Autodesk Inventor part; units mm, degrees
(part 4 of 4)
sketch "Эскиз15" plane through (0, 0, 5) normal (0, 0, 1) x (1, 0, 0)
  circle A0 centre (-47.4326, -62.0164) radius 1.6 projected
  circle A1 centre (-37.1084, -66.6437) radius 1.6 projected
  circle A2 centre (-32.4811, -56.3196) radius 1.6 projected
  circle A3 centre (-39.9568, -59.168) radius 2.5 projected
  circle A4 centre (-42.8052, -51.6922) radius 1.6 projected
  arc A5 (-41.4259, -46.9885) -> (-28.2942, -62.9735) centre (-39.9568, -59.168) ccw projected
  line L0 (-28.085, -62.2597) -> (-28.2942, -62.9735) projected
  line L1 (-27.9195, -61.5344) -> (-28.085, -62.2597) projected
  line L2 (-27.7675, -61.2078) -> (-27.9195, -61.5344) projected
  line L3 (-27.6559, -61.0885) -> (-27.7675, -61.2078) projected
  line L4 (-27.5511, -61.0052) -> (-27.6559, -61.0885) projected
  line L5 (-27.4498, -60.9413) -> (-27.5511, -61.0052) projected
  line L6 (-27.3508, -60.8903) -> (-27.4498, -60.9413) projected
  line L7 (-27.1571, -60.815) -> (-27.3508, -60.8903) projected
  line L8 (-26.9672, -60.7651) -> (-27.1571, -60.815) projected
  line L9 (-26.78, -60.734) -> (-26.9672, -60.7651) projected
  line L10 (-26.5947, -60.7178) -> (-26.78, -60.734) projected
  line L11 (-26.2284, -60.7215) -> (-26.5947, -60.7178) projected
  line L12 (-25.8656, -60.755) -> (-26.2284, -60.7215) projected
  line L13 (-25.4958, -60.7256) -> (-25.8656, -60.755) projected
  line L14 (-25.1221, -60.6541) -> (-25.4958, -60.7256) projected
  line L15 (-24.7463, -60.5502) -> (-25.1221, -60.6541) projected
  line L16 (-24.3693, -60.4182) -> (-24.7463, -60.5502) projected
  line L17 (-23.9923, -60.2602) -> (-24.3693, -60.4182) projected
  line L18 (-23.616, -60.0777) -> (-23.9923, -60.2602) projected
  line L19 (-23.2412, -59.8717) -> (-23.616, -60.0777) projected
  line L20 (-22.8687, -59.6431) -> (-23.2412, -59.8717) projected
  line L21 (-22.4992, -59.3924) -> (-22.8687, -59.6431) projected
  line L22 (-22.2246, -59.1902) -> (-22.4992, -59.3924) projected
  line L23 (-22.3522, -57.0445) -> (-22.2246, -59.1902) projected
  line L24 (-22.6489, -56.8763) -> (-22.3522, -57.0445) projected
  line L25 (-23.0454, -56.6711) -> (-22.6489, -56.8763) projected
  line L26 (-23.4424, -56.4882) -> (-23.0454, -56.6711) projected
  line L27 (-23.839, -56.3281) -> (-23.4424, -56.4882) projected
  line L28 (-24.2343, -56.1915) -> (-23.839, -56.3281) projected
  line L29 (-24.6274, -56.0793) -> (-24.2343, -56.1915) projected
  line L30 (-25.0173, -55.9929) -> (-24.6274, -56.0793) projected
  line L31 (-25.4028, -55.9343) -> (-25.0173, -55.9929) projected
  line L32 (-25.7823, -55.9075) -> (-25.4028, -55.9343) projected
  line L33 (-26.153, -55.9222) -> (-25.7823, -55.9075) projected
  line L34 (-26.5093, -55.9985) -> (-26.153, -55.9222) projected
  line L35 (-26.8725, -56.0456) -> (-26.5093, -55.9985) projected
  line L36 (-27.0584, -56.0515) -> (-26.8725, -56.0456) projected
  line L37 (-27.248, -56.0427) -> (-27.0584, -56.0515) projected
  line L38 (-27.4425, -56.0157) -> (-27.248, -56.0427) projected
  line L39 (-27.6437, -55.9639) -> (-27.4425, -56.0157) projected
  line L40 (-27.7481, -55.925) -> (-27.6437, -55.9639) projected
  line L41 (-27.8563, -55.8736) -> (-27.7481, -55.925) projected
  line L42 (-27.9702, -55.8032) -> (-27.8563, -55.8736) projected
  line L43 (-28.0951, -55.698) -> (-27.9702, -55.8032) projected
  line L44 (-28.2847, -55.3917) -> (-28.0951, -55.698) projected
  line L45 (-28.5351, -54.6912) -> (-28.2847, -55.3917) projected
  line L46 (-28.8274, -54.0071) -> (-28.5351, -54.6912) projected
  line L47 (-28.8965, -53.6536) -> (-28.8274, -54.0071) projected
  line L48 (-28.8763, -53.4914) -> (-28.8965, -53.6536) projected
  line L49 (-28.8405, -53.3624) -> (-28.8763, -53.4914) projected
  line L50 (-28.7962, -53.2512) -> (-28.8405, -53.3624) projected
  line L51 (-28.746, -53.1517) -> (-28.7962, -53.2512) projected
  line L52 (-28.6335, -52.977) -> (-28.746, -53.1517) projected
  line L53 (-28.5092, -52.825) -> (-28.6335, -52.977) projected
  line L54 (-28.3761, -52.6897) -> (-28.5092, -52.825) projected
  line L55 (-28.2357, -52.5677) -> (-28.3761, -52.6897) projected
  line L56 (-27.9372, -52.3554) -> (-28.2357, -52.5677) projected
  line L57 (-27.624, -52.1693) -> (-27.9372, -52.3554) projected
  line L58 (-27.3421, -51.9282) -> (-27.624, -52.1693) projected
  line L59 (-27.0818, -51.6507) -> (-27.3421, -51.9282) projected
  line L60 (-26.8388, -51.3457) -> (-27.0818, -51.6507) projected
  line L61 (-26.6114, -51.0173) -> (-26.8388, -51.3457) projected
  line L62 (-26.3993, -50.6679) -> (-26.6114, -51.0173) projected
  line L63 (-26.2021, -50.2991) -> (-26.3993, -50.6679) projected
  line L64 (-26.02, -49.9121) -> (-26.2021, -50.2991) projected
  line L65 (-25.853, -49.5082) -> (-26.02, -49.9121) projected
  line L66 (-25.7014, -49.0882) -> (-25.853, -49.5082) projected
  line L67 (-25.5981, -48.7632) -> (-25.7014, -49.0882) projected
  line L68 (-25.5981, -48.7632) -> (-26.9625, -47.1023) projected
  line L69 (-27.3014, -47.1406) -> (-26.9625, -47.1023) projected
  line L70 (-27.7429, -47.2077) -> (-27.3014, -47.1406) projected
  line L71 (-28.1715, -47.2931) -> (-27.7429, -47.2077) projected
  line L72 (-28.5864, -47.3967) -> (-28.1715, -47.2931) projected
  line L73 (-28.9865, -47.5185) -> (-28.5864, -47.3967) projected
  line L74 (-29.3705, -47.6588) -> (-28.9865, -47.5185) projected
  line L75 (-29.7368, -47.818) -> (-29.3705, -47.6588) projected
  line L76 (-30.0831, -47.9973) -> (-29.7368, -47.818) projected
  line L77 (-30.4059, -48.1987) -> (-30.0831, -47.9973) projected
  line L78 (-30.6971, -48.4284) -> (-30.4059, -48.1987) projected
  line L79 (-30.9405, -48.6995) -> (-30.6971, -48.4284) projected
  line L80 (-31.2067, -48.9511) -> (-30.9405, -48.6995) projected
  line L81 (-31.3536, -49.0652) -> (-31.2067, -48.9511) projected
  line L82 (-31.5122, -49.1695) -> (-31.3536, -49.0652) projected
  line L83 (-31.6854, -49.262) -> (-31.5122, -49.1695) projected
  line L84 (-31.8786, -49.3384) -> (-31.6854, -49.262) projected
  line L85 (-31.986, -49.3683) -> (-31.8786, -49.3384) projected
  line L86 (-32.1037, -49.3902) -> (-31.986, -49.3683) projected
  line L87 (-32.2372, -49.4003) -> (-32.1037, -49.3902) projected
  line L88 (-32.4002, -49.3886) -> (-32.2372, -49.4003) projected
  line L89 (-32.7336, -49.2522) -> (-32.4002, -49.3886) projected
  line L90 (-33.3479, -48.8326) -> (-32.7336, -49.2522) projected
  line L91 (-33.9864, -48.4511) -> (-33.3479, -48.8326) projected
  line L92 (-34.2501, -48.2056) -> (-33.9864, -48.4511) projected
  line L93 (-34.3291, -48.0626) -> (-34.2501, -48.2056) projected
  line L94 (-34.376, -47.9372) -> (-34.3291, -48.0626) projected
  line L95 (-34.4055, -47.8211) -> (-34.376, -47.9372) projected
  line L96 (-34.4234, -47.7112) -> (-34.4055, -47.8211) projected
  line L97 (-34.4351, -47.5037) -> (-34.4234, -47.7112) projected
  line L98 (-34.4238, -47.3077) -> (-34.4351, -47.5037) projected
  line L99 (-34.3956, -47.12) -> (-34.4238, -47.3077) projected
  line L100 (-34.3538, -46.9387) -> (-34.3956, -47.12) projected
  line L101 (-34.237, -46.5916) -> (-34.3538, -46.9387) projected
  line L102 (-34.0931, -46.2568) -> (-34.237, -46.5916) projected
  line L103 (-34.0067, -45.8961) -> (-34.0931, -46.2568) projected
  line L104 (-33.9593, -45.5186) -> (-34.0067, -45.8961) projected
  line L105 (-33.9419, -45.129) -> (-33.9593, -45.5186) projected
  line L106 (-33.951, -44.7298) -> (-33.9419, -45.129) projected
  line L107 (-33.9848, -44.3224) -> (-33.951, -44.7298) projected
  line L108 (-34.0421, -43.9081) -> (-33.9848, -44.3224) projected
  line L109 (-34.1221, -43.488) -> (-34.0421, -43.9081) projected
  line L110 (-34.2244, -43.063) -> (-34.1221, -43.488) projected
  line L111 (-34.3487, -42.6342) -> (-34.2244, -43.063) projected
  line L112 (-34.4561, -42.3105) -> (-34.3487, -42.6342) projected
  line L113 (-36.5363, -41.7688) -> (-34.4561, -42.3105) projected
  line L114 (-36.7879, -41.999) -> (-36.5363, -41.7688) projected
  line L115 (-37.1056, -42.3127) -> (-36.7879, -41.999) projected
  line L116 (-37.4022, -42.6338) -> (-37.1056, -42.3127) projected
  line L117 (-37.677, -42.9614) -> (-37.4022, -42.6338) projected
  line L118 (-37.9291, -43.2952) -> (-37.677, -42.9614) projected
  line L119 (-38.1573, -43.6344) -> (-37.9291, -43.2952) projected
  line L120 (-38.36, -43.9785) -> (-38.1573, -43.6344) projected
  line L121 (-38.5348, -44.327) -> (-38.36, -43.9785) projected
  line L122 (-38.6775, -44.6797) -> (-38.5348, -44.327) projected
  line L123 (-38.7781, -45.0367) -> (-38.6775, -44.6797) projected
  line L124 (-38.8157, -45.3992) -> (-38.7781, -45.0367) projected
  line L125 (-38.8831, -45.7592) -> (-38.8157, -45.3992) projected
  line L126 (-38.935, -45.9378) -> (-38.8831, -45.7592) projected
  line L127 (-39.0019, -46.1155) -> (-38.935, -45.9378) projected
  line L128 (-39.0877, -46.292) -> (-39.0019, -46.1155) projected
  line L129 (-39.1991, -46.4674) -> (-39.0877, -46.292) projected
  line L130 (-39.2684, -46.5547) -> (-39.1991, -46.4674) projected
  line L131 (-39.3507, -46.6417) -> (-39.2684, -46.5547) projected
  line L132 (-39.4528, -46.7283) -> (-39.3507, -46.6417) projected
  line L133 (-39.5916, -46.8146) -> (-39.4528, -46.7283) projected
  line L134 (-39.9414, -46.9002) -> (-39.5916, -46.8146) projected
  line L135 (-40.685, -46.9219) -> (-39.9414, -46.9002) projected
  line L136 (-41.4259, -46.9885) -> (-40.685, -46.9219) projected
  circle A6 centre (-39.9568, -59.168) radius 12.2678
  point P0 (0, 0)
  point P1 (-32.7336, -49.2522)
  point P2 (-28.8274, -54.0071)
  point P3 (-33.9864, -48.4511)
  constraints: 1 centre point, 1 concentric
extrude "Выдавливание14" cut sketch "Эскиз15" against normal blind 10 contours L134 L133 L132 L131 L130 L129 L128 L127 L126 L125 L124 L123 L122 L121 L120 L119 L118 L117 L116 L115 L114 L113 L112 L111 L110 L109 L108 L107 L106 L105 L104 L103 L102 L101 L100 L99 L98 L97 L96 L95 L94 L93 L92 A6 | A6 L44 L43 L42 L41 L40 L39 L38 L37 L36 L35 L34 L33 L32 L31 L30 L29 L28 L27 L26 L25 L24 L23 L22 L21 L20 L19 L18 L17 L16 L15 L14 L13 L12 L11 L10 L9 L8 L7 L6 L5 L4 L3 L2 | L89 L88 L87 L86 L85 L84 L83 L82 L81 L80 L79 L78 L77 L76 L75 L74 L73 L72 L71 L70 L69 L68 L67 L66 L65 L64 L63 L62 L61 L60 L59 L58 L57 L56 L55 L54 L53 L52 L51 L50 L49 L48 L47 A6
sketch "Эскиз16" plane through (0, 0, 5) normal (0, 0, 1) x (1, 0, 0)
  arc A0 (-16.2314, -59.2639) -> (-22.5655, -38.0436) centre (-14.0874, -47.0684) ccw projected
  arc A1 (-22.5655, -38.0436) -> (-25.2878, -36.7337) centre (-28.6703, -47.2467) ccw projected
  arc A2 (-25.2878, -36.7337) -> (-25.9966, -37.559) centre (-14.0874, -47.0684) ccw projected
  arc A3 (-25.9966, -37.559) -> (-24.2901, -40.052) centre (-16.1157, -32.6262) ccw projected
  arc A4 (-24.2901, -40.052) -> (-24.7647, -40.7978) centre (-14.0874, -47.0684) ccw projected
  arc A5 (-24.7647, -40.7978) -> (-27.7458, -40.3078) centre (-28.0294, -51.3479) ccw projected
  arc A6 (-27.7458, -40.3078) -> (-28.1933, -41.2994) centre (-14.0874, -47.0684) ccw projected
  arc A7 (-28.1933, -41.2994) -> (-25.8536, -43.2107) centre (-20.1024, -33.7826) ccw projected
  arc A8 (-25.8536, -43.2107) -> (-26.0988, -44.0599) centre (-14.0874, -47.0684) ccw projected
  arc A9 (-26.0988, -44.0599) -> (-29.0972, -44.4297) centre (-26.2589, -55.1025) ccw projected
  arc A10 (-29.0972, -44.4297) -> (-29.2472, -45.5072) centre (-14.0874, -47.0684) ccw projected
  arc A11 (-29.2472, -45.5072) -> (-26.4639, -46.6819) centre (-23.6018, -36.0154) ccw projected
  arc A12 (-26.4639, -46.6819) -> (-26.4599, -47.5658) centre (-14.0874, -47.0684) ccw projected
  arc A13 (-26.4599, -47.5658) -> (-29.2326, -48.7653) centre (-23.5025, -58.2062) ccw projected
  arc A14 (-29.2326, -48.7653) -> (-29.073, -49.8415) centre (-14.0874, -47.0684) ccw projected
  arc A15 (-29.073, -49.8415) -> (-26.0714, -50.1844) centre (-26.3304, -39.1437) ccw projected
  arc A16 (-26.0714, -50.1844) -> (-25.8186, -51.0314) centre (-14.0874, -47.0684) ccw projected
  arc A17 (-25.8186, -51.0314) -> (-28.1411, -52.9635) centre (-19.9832, -60.4075) ccw projected
  arc A18 (-28.1411, -52.9635) -> (-27.6847, -53.9511) centre (-14.0874, -47.0684) ccw projected
  arc A19 (-27.6847, -53.9511) -> (-24.7081, -53.4345) centre (-28.0671, -42.9139) ccw projected
  arc A20 (-24.7081, -53.4345) -> (-24.2269, -54.1759) centre (-14.0874, -47.0684) ccw projected
  arc A21 (-24.2269, -54.1759) -> (-25.911, -56.6841) centre (-15.9863, -61.5283) ccw projected
  arc A22 (-25.911, -56.6841) -> (-25.1949, -57.5031) centre (-14.0874, -47.0684) ccw projected
  arc A23 (-25.1949, -57.5031) -> (-22.4844, -56.1688) centre (-28.6713, -47.0208) ccw projected
  arc A24 (-22.4844, -56.1688) -> (-21.8138, -56.7447) centre (-14.0874, -47.0684) ccw projected
  arc A25 (-21.8138, -56.7447) -> (-22.723, -59.6257) centre (-11.8356, -61.4775) ccw projected
  arc A26 (-22.723, -59.6257) -> (-21.8052, -60.2097) centre (-14.0874, -47.0684) ccw projected
  arc A27 (-21.8052, -60.2097) -> (-19.5804, -58.1659) centre (-28.094, -51.1315) ccw projected
  arc A28 (-19.5804, -58.1659) -> (-18.7747, -58.5295) centre (-14.0874, -47.0684) ccw projected
  arc A29 (-18.7747, -58.5295) -> (-18.8354, -61.5499) centre (-7.8673, -60.2595) ccw projected
  arc A30 (-18.8354, -61.5499) -> (-17.7902, -61.8518) centre (-14.0874, -47.0684) ccw projected
  arc A31 (-17.7902, -61.8518) -> (-16.2314, -59.2639) centre (-26.3819, -54.913) ccw projected
  circle A32 centre (-9.9505, -53.9158) radius 1.6 projected
  circle A33 centre (-20.9347, -51.2053) radius 1.6 projected
  circle A34 centre (-18.2243, -40.2211) radius 1.6 projected
  circle A35 centre (-7.2401, -42.9315) radius 1.6 projected
  circle A36 centre (-14.0874, -47.0684) radius 2.5 projected
  arc A37 (-27.9195, -61.5344) -> (-28.2847, -55.3917) centre (-39.9568, -59.168) ccw projected
  line L0 (-28.5351, -54.6912) -> (-28.2847, -55.3917) projected
  line L1 (-28.8274, -54.0071) -> (-28.5351, -54.6912) projected
  arc A38 (-28.8274, -54.0071) -> (-32.7336, -49.2522) centre (-39.9568, -59.168) ccw projected
  line L2 (-33.3479, -48.8326) -> (-32.7336, -49.2522) projected
  line L3 (-33.9864, -48.4511) -> (-33.3479, -48.8326) projected
  arc A39 (-33.9864, -48.4511) -> (-39.9414, -46.9002) centre (-39.9568, -59.168) ccw projected
  line L4 (-40.685, -46.9219) -> (-39.9414, -46.9002) projected
  line L5 (-41.4259, -46.9885) -> (-40.685, -46.9219) projected
  arc A40 (-41.4259, -46.9885) -> (-28.2942, -62.9735) centre (-39.9568, -59.168) ccw projected
  line L6 (-28.085, -62.2597) -> (-28.2942, -62.9735) projected
  line L7 (-27.9195, -61.5344) -> (-28.085, -62.2597) projected
  circle A41 centre (-47.4326, -62.0164) radius 1.6 projected
  circle A42 centre (-37.1084, -66.6437) radius 1.6 projected
  circle A43 centre (-32.4811, -56.3196) radius 1.6 projected
  circle A44 centre (-39.9568, -59.168) radius 2.5 projected
  circle A45 centre (-42.8052, -51.6922) radius 1.6 projected
  arc A46 (-28.8099, -64.5599) -> (-28.4537, -63.7509) centre (-39.9568, -59.168) ccw
  arc A47 (-28.4537, -63.7509) -> (-25.4328, -63.7842) centre (-26.8229, -52.8283) ccw
  arc A48 (-25.4328, -63.7842) -> (-25.1404, -62.7363) centre (-39.9568, -59.168) ccw
  arc A49 (-25.1404, -62.7363) -> (-27.7424, -61.201) centre (-32.0008, -71.3907) ccw
  arc A50 (-27.7424, -61.201) -> (-27.6284, -60.3245) centre (-39.9568, -59.168) ccw
  arc A51 (-27.6284, -60.3245) -> (-24.7206, -59.5053) centre (-29.141, -49.3848) ccw
  arc A52 (-24.7206, -59.5053) -> (-24.7353, -58.4175) centre (-39.9568, -59.168) ccw
  arc A53 (-24.7353, -58.4175) -> (-27.6644, -57.6775) centre (-28.8796, -68.6541) ccw
  arc A54 (-27.6644, -57.6775) -> (-27.802, -56.8043) centre (-39.9568, -59.168) ccw
  arc A55 (-27.802, -56.8043) -> (-25.2427, -55.1991) centre (-32.3353, -46.7339) ccw
  arc A56 (-25.2427, -55.1991) -> (-25.5633, -54.1595) centre (-39.9568, -59.168) ccw
  arc A57 (-25.5633, -54.1595) -> (-28.5822, -54.2747) centre (-26.6557, -65.1491) ccw
  arc A58 (-28.5822, -54.2747) -> (-28.9603, -53.4757) centre (-39.9568, -59.168) ccw
  arc A59 (-28.9603, -53.4757) -> (-26.9569, -51.2144) centre (-36.1472, -45.0904) ccw
  arc A60 (-26.9569, -51.2144) -> (-27.5574, -50.3073) centre (-39.9568, -59.168) ccw
  arc A61 (-27.5574, -50.3073) -> (-30.4216, -51.2683) centre (-25.5094, -61.1594) ccw
  arc A62 (-30.4216, -51.2683) -> (-31.0094, -50.6082) centre (-39.9568, -59.168) ccw
  arc A63 (-31.0094, -50.6082) -> (-29.7243, -47.8741) centre (-40.2676, -44.5873) ccw
  arc A64 (-29.7243, -47.8741) -> (-30.556, -47.1729) centre (-39.9568, -59.168) ccw
  arc A65 (-30.556, -47.1729) -> (-33.0334, -48.9019) centre (-25.5336, -57.0085) ccw
  arc A66 (-33.0334, -48.9019) -> (-33.7834, -48.4341) centre (-39.9568, -59.168) ccw
  arc A67 (-33.7834, -48.4341) -> (-33.3206, -45.4487) centre (-44.3629, -45.2655) ccw
  arc A68 (-33.3206, -45.4487) -> (-34.3163, -45.0102) centre (-39.9568, -59.168) ccw
  arc A69 (-34.3163, -45.0102) -> (-36.2062, -47.3672) centre (-26.7263, -53.0325) ccw
  arc A70 (-36.2062, -47.3672) -> (-37.0576, -47.1297) centre (-39.9568, -59.168) ccw
  arc A71 (-37.0576, -47.1297) -> (-37.4546, -44.1348) centre (-48.1012, -47.07) ccw
  arc A72 (-37.4546, -44.1348) -> (-38.5334, -43.9946) centre (-39.9568, -59.168) ccw
  arc A73 (-38.5334, -43.9946) -> (-39.6828, -46.7885) centre (-28.9908, -49.5535) ccw
  arc A74 (-39.6828, -46.7885) -> (-40.5666, -46.8005) centre (-39.9568, -59.168) ccw
  arc A75 (-40.5666, -46.8005) -> (-41.7913, -44.0388) centre (-51.1797, -49.8545) ccw
  arc A76 (-41.7913, -44.0388) -> (-42.8659, -44.2082) centre (-39.9568, -59.168) ccw
  arc A77 (-42.8659, -44.2082) -> (-43.1816, -47.2128) centre (-32.1437, -46.8535) ccw
  arc A78 (-43.1816, -47.2128) -> (-44.0262, -47.4733) centre (-39.9568, -59.168) ccw
  circle A79 centre (-39.9568, -59.168) radius 12.3825
  point P0 (0, 0)
  point P1 (-27.7424, -61.201)
  point P2 (-28.4537, -63.7509)
  point P3 (-27.6644, -57.6775)
  point P4 (-27.6284, -60.3245)
  point P5 (-28.5822, -54.2747)
  point P6 (-27.802, -56.8043)
  point P7 (-30.4216, -51.2683)
  point P8 (-28.9603, -53.4757)
  point P9 (-31.0094, -50.6082)
  point P10 (-36.2062, -47.3672)
  point P11 (-33.7834, -48.4341)
  point P12 (-37.0576, -47.1297)
  point P13 (-43.1816, -47.2128)
  point P14 (-28.8099, -64.5599)
  point P15 (-28.4537, -63.7509)
  point P16 (-27.7424, -61.201)
  point P17 (-27.6284, -60.3245)
  point P18 (-27.6644, -57.6775)
  point P19 (-27.802, -56.8043)
  point P20 (-28.5822, -54.2747)
  point P21 (-28.9603, -53.4757)
  point P22 (-30.4216, -51.2683)
  point P23 (-31.0094, -50.6082)
  point P24 (-33.7834, -48.4341)
  point P25 (-36.2062, -47.3672)
  point P26 (-37.0576, -47.1297)
  point P27 (-43.1816, -47.2128)
  point P28 (-44.0262, -47.4733)
  constraints: 66 point on circle, 33 centre point, 2 other
extrude "Выдавливание15" add sketch "Эскиз16" against normal up to surface (5 mm away) contours A79 A49 A48 A47 | A77 A76 A75 A79 | A79 A53 A52 A51 | A73 A72 A71 A79 | A79 A57 A56 A55 | A69 A68 A67 A79 | A79 A61 A60 A59 | A65 A64 A63 A79
sketch "Эскиз17" plane through (0, 0, 5) normal (0, 0, 1) x (1, 0, 0)
  circle A0 centre (-39.9568, -59.168) radius 2.5 projected
  circle A1 centre (-20.698, -37.4863) radius 2.5 projected
  line L0 (-20.698, -37.4863) -> (-39.9568, -59.168)
  line L1 (-30.3274, -48.3271) -> (-82.2818, -2.1785)
  point P0 (0, 0)
  constraints: 4 end point, 1 midpoint, 1 perpendicular
sketch "Эскиз18" plane through (0, 0, 5) normal (0, 0, 1) x (1, 0, 0)
  line L0 (-68.9905, -23.1935) -> (-67.6185, -42.7187) projected
  arc A0 (-43.1816, -47.2128) -> (-28.4537, -63.7509) centre (-39.9568, -59.168) ccw projected
  line L1 (-67.7849, -22.278) -> (-74.8978, -22.7778)
  line L2 (-66.4131, -41.803) -> (-65.4189, -44.6336)
  line L3 (-71.6748, -50.2404) -> (-73.2914, -45.6377)
  line L4 (-73.2914, -45.6377) -> (-74.8978, -22.7778)
  ellipse E0 centre (-53.6547, -42.8166) end of major axis (-126.4395, -125.8166) minor radius 2.3654 (-52.7653, -45.3897) -> (-36.6582, -26.9425) ccw
  line L5 (-67.7849, -22.278) -> (-66.4131, -41.803)
  line L6 (-48.2799, -50) -> (-65.4189, -44.6336)
  line L7 (-48.6356, -68) -> (-71.6748, -50.2404)
  point P0 (0, 0)
  point P1 (-60.3958, -58.9347)
  point P2 (-65.4187, -44.6336)
  constraints: 14 end point, 2 parallel, 2 point on circle, 2 point on line, 1 perpendicular, 7 other
extrude "Выдавливание16" add sketch "Эскиз18" against normal up to surface (5 mm away)
fillet "Сопряжение1" [suppressed]
sketch "Эскиз19" plane through (0, 0, 5) normal (0, 0, 1) x (1, 0, 0)
  arc A0 (-38.5334, -43.9946) -> (-39.6828, -46.7885) centre (-28.9908, -49.5535) ccw projected
  arc A1 (-39.6828, -46.7885) -> (-40.5666, -46.8005) centre (-39.9568, -59.168) ccw projected
  arc A2 (-40.5666, -46.8005) -> (-41.7913, -44.0388) centre (-51.1797, -49.8545) ccw projected
  arc A3 (-41.7913, -44.0388) -> (-42.8659, -44.2082) centre (-39.9568, -59.168) ccw projected
  arc A4 (-42.8659, -44.2082) -> (-43.1816, -47.2128) centre (-32.1437, -46.8535) ccw projected
  arc A5 (-43.1816, -47.2128) -> (-48.2799, -50) centre (-39.9568, -59.168) ccw projected
  arc A6 (-28.4537, -63.7509) -> (-25.4328, -63.7842) centre (-26.8229, -52.8283) ccw projected
  arc A7 (-25.4328, -63.7842) -> (-25.1404, -62.7363) centre (-39.9568, -59.168) ccw projected
  arc A8 (-25.1404, -62.7363) -> (-27.7424, -61.201) centre (-32.0008, -71.3907) ccw projected
  arc A9 (-27.7424, -61.201) -> (-27.6284, -60.3245) centre (-39.9568, -59.168) ccw projected
  arc A10 (-27.6284, -60.3245) -> (-24.7206, -59.5053) centre (-29.141, -49.3848) ccw projected
  arc A11 (-24.7206, -59.5053) -> (-24.7353, -58.4175) centre (-39.9568, -59.168) ccw projected
  arc A12 (-24.7353, -58.4175) -> (-27.6644, -57.6775) centre (-28.8796, -68.6541) ccw projected
  arc A13 (-27.6644, -57.6775) -> (-27.802, -56.8043) centre (-39.9568, -59.168) ccw projected
  arc A14 (-27.802, -56.8043) -> (-25.2427, -55.1991) centre (-32.3353, -46.7339) ccw projected
  arc A15 (-25.2427, -55.1991) -> (-25.5633, -54.1595) centre (-39.9568, -59.168) ccw projected
  arc A16 (-25.5633, -54.1595) -> (-28.5822, -54.2747) centre (-26.6557, -65.1491) ccw projected
  arc A17 (-28.5822, -54.2747) -> (-28.9603, -53.4757) centre (-39.9568, -59.168) ccw projected
  arc A18 (-28.9603, -53.4757) -> (-26.9569, -51.2144) centre (-36.1472, -45.0904) ccw projected
  arc A19 (-26.9569, -51.2144) -> (-27.5574, -50.3073) centre (-39.9568, -59.168) ccw projected
  arc A20 (-27.5574, -50.3073) -> (-30.4216, -51.2683) centre (-25.5094, -61.1594) ccw projected
  arc A21 (-30.4216, -51.2683) -> (-31.0094, -50.6082) centre (-39.9568, -59.168) ccw projected
  arc A22 (-31.0094, -50.6082) -> (-29.7243, -47.8741) centre (-40.2676, -44.5873) ccw projected
  arc A23 (-29.7243, -47.8741) -> (-30.556, -47.1729) centre (-39.9568, -59.168) ccw projected
  arc A24 (-30.556, -47.1729) -> (-33.0334, -48.9019) centre (-25.5336, -57.0085) ccw projected
  arc A25 (-33.0334, -48.9019) -> (-33.7834, -48.4341) centre (-39.9568, -59.168) ccw projected
  arc A26 (-33.7834, -48.4341) -> (-33.3206, -45.4487) centre (-44.3629, -45.2655) ccw projected
  arc A27 (-33.3206, -45.4487) -> (-34.3163, -45.0102) centre (-39.9568, -59.168) ccw projected
  arc A28 (-34.3163, -45.0102) -> (-36.2062, -47.3672) centre (-26.7263, -53.0325) ccw projected
  arc A29 (-36.2062, -47.3672) -> (-37.0576, -47.1297) centre (-39.9568, -59.168) ccw projected
  arc A30 (-37.0576, -47.1297) -> (-37.4546, -44.1348) centre (-48.1012, -47.07) ccw projected
  arc A31 (-37.4546, -44.1348) -> (-38.5334, -43.9946) centre (-39.9568, -59.168) ccw projected
  circle A32 centre (-47.4326, -62.0164) radius 1.6 projected
  circle A33 centre (-37.1084, -66.6437) radius 1.6 projected
  circle A34 centre (-32.4811, -56.3196) radius 1.6 projected
  circle A35 centre (-39.9568, -59.168) radius 2.5 projected
  circle A36 centre (-42.8052, -51.6922) radius 1.6 projected
  circle A37 centre (-17.9668, -53.9582) radius 1.6
  circle A38 centre (-10.9861, -57.8658) radius 2.5
  circle A39 centre (-14.8937, -64.8466) radius 1.6
  circle A40 centre (-4.0053, -61.7734) radius 1.6
  circle A41 centre (-7.0785, -50.8851) radius 1.6
  arc A42 (-22.6473, -62.0301) -> (-1.343, -65.6336) centre (-10.9861, -57.8658) ccw
  arc A43 (-12.9434, -42.752) -> (-13.4484, -45.7306) centre (-2.4099, -46.07) ccw
  arc A44 (-10.8126, -45.4845) -> (-11.8602, -42.6509) centre (-21.5975, -47.8613) ccw
  arc A45 (-23.266, -59.4561) -> (-25.9217, -60.8964) centre (-19.3786, -69.7931) ccw
  arc A46 (-25.6675, -61.9541) -> (-22.6473, -62.0301) centre (-23.8823, -51.0556) ccw
  line L0 (-48.2799, -50) -> (-65.4189, -44.6336) projected
  line L1 (-65.4189, -44.6336) -> (-66.4131, -41.803) projected
  line L2 (-66.4131, -41.803) -> (-67.7849, -22.278) projected
  line L3 (-67.7849, -22.278) -> (-74.8978, -22.7778) projected
  line L4 (-74.8978, -22.7778) -> (-73.2914, -45.6377) projected
  line L5 (-73.2914, -45.6377) -> (-71.6748, -50.2404) projected
  line L6 (-71.6748, -50.2404) -> (-48.6356, -68) projected
  arc A47 (-48.6356, -68) -> (-28.4537, -63.7509) centre (-39.9568, -59.168) ccw projected
  point P0 (0, 0)
  constraints: 10 centre point, 10 point on circle, 29 other
sketch "Эскиз20" plane through (0, 0, 5) normal (0, 0, 1) x (1, 0, 0)
  arc A0 (-38.5334, -43.9946) -> (-39.6828, -46.7885) centre (-28.9908, -49.5535) ccw projected
  arc A1 (-39.6828, -46.7885) -> (-40.5666, -46.8005) centre (-39.9568, -59.168) ccw projected
  arc A2 (-40.5666, -46.8005) -> (-41.7913, -44.0388) centre (-51.1797, -49.8545) ccw projected
  arc A3 (-41.7913, -44.0388) -> (-42.8659, -44.2082) centre (-39.9568, -59.168) ccw projected
  arc A4 (-42.8659, -44.2082) -> (-43.1816, -47.2128) centre (-32.1437, -46.8535) ccw projected
  arc A5 (-43.1816, -47.2128) -> (-48.2799, -50) centre (-39.9568, -59.168) ccw projected
  line L0 (-48.2799, -50) -> (-65.4189, -44.6336) projected
  line L1 (-65.4189, -44.6336) -> (-66.4131, -41.803) projected
  line L2 (-66.4131, -41.803) -> (-67.7849, -22.278) projected
  line L3 (-67.7849, -22.278) -> (-74.8978, -22.7778) projected
  line L4 (-74.8978, -22.7778) -> (-73.2914, -45.6377) projected
  line L5 (-73.2914, -45.6377) -> (-71.6748, -50.2404) projected
  line L6 (-71.6748, -50.2404) -> (-48.6356, -68) projected
  arc A6 (-48.6356, -68) -> (-28.4537, -63.7509) centre (-39.9568, -59.168) ccw projected
  arc A7 (-28.4537, -63.7509) -> (-25.4328, -63.7842) centre (-26.8229, -52.8283) ccw projected
  arc A8 (-25.4328, -63.7842) -> (-25.1404, -62.7363) centre (-39.9568, -59.168) ccw projected
  arc A9 (-25.1404, -62.7363) -> (-27.7424, -61.201) centre (-32.0008, -71.3907) ccw projected
  arc A10 (-27.7424, -61.201) -> (-27.6284, -60.3245) centre (-39.9568, -59.168) ccw projected
  arc A11 (-27.6284, -60.3245) -> (-24.7206, -59.5053) centre (-29.141, -49.3848) ccw projected
  arc A12 (-24.7206, -59.5053) -> (-24.7353, -58.4175) centre (-39.9568, -59.168) ccw projected
  arc A13 (-24.7353, -58.4175) -> (-27.6644, -57.6775) centre (-28.8796, -68.6541) ccw projected
  arc A14 (-27.6644, -57.6775) -> (-27.802, -56.8043) centre (-39.9568, -59.168) ccw projected
  arc A15 (-27.802, -56.8043) -> (-25.2427, -55.1991) centre (-32.3353, -46.7339) ccw projected
  arc A16 (-25.2427, -55.1991) -> (-25.5633, -54.1595) centre (-39.9568, -59.168) ccw projected
  arc A17 (-25.5633, -54.1595) -> (-28.5822, -54.2747) centre (-26.6557, -65.1491) ccw projected
  arc A18 (-28.5822, -54.2747) -> (-28.9603, -53.4757) centre (-39.9568, -59.168) ccw projected
  arc A19 (-28.9603, -53.4757) -> (-26.9569, -51.2144) centre (-36.1472, -45.0904) ccw projected
  arc A20 (-26.9569, -51.2144) -> (-27.5574, -50.3073) centre (-39.9568, -59.168) ccw projected
  arc A21 (-27.5574, -50.3073) -> (-30.4216, -51.2683) centre (-25.5094, -61.1594) ccw projected
  arc A22 (-30.4216, -51.2683) -> (-31.0094, -50.6082) centre (-39.9568, -59.168) ccw projected
  arc A23 (-31.0094, -50.6082) -> (-29.7243, -47.8741) centre (-40.2676, -44.5873) ccw projected
  arc A24 (-29.7243, -47.8741) -> (-30.556, -47.1729) centre (-39.9568, -59.168) ccw projected
  arc A25 (-30.556, -47.1729) -> (-33.0334, -48.9019) centre (-25.5336, -57.0085) ccw projected
  arc A26 (-33.0334, -48.9019) -> (-33.7834, -48.4341) centre (-39.9568, -59.168) ccw projected
  arc A27 (-33.7834, -48.4341) -> (-33.3206, -45.4487) centre (-44.3629, -45.2655) ccw projected
  arc A28 (-33.3206, -45.4487) -> (-34.3163, -45.0102) centre (-39.9568, -59.168) ccw projected
  arc A29 (-34.3163, -45.0102) -> (-36.2062, -47.3672) centre (-26.7263, -53.0325) ccw projected
  arc A30 (-36.2062, -47.3672) -> (-37.0576, -47.1297) centre (-39.9568, -59.168) ccw projected
  arc A31 (-37.0576, -47.1297) -> (-37.4546, -44.1348) centre (-48.1012, -47.07) ccw projected
  arc A32 (-37.4546, -44.1348) -> (-38.5334, -43.9946) centre (-39.9568, -59.168) ccw projected
  circle A33 centre (-47.4326, -62.0164) radius 1.6 projected
  circle A34 centre (-37.1084, -66.6437) radius 1.6 projected
  circle A35 centre (-32.4811, -56.3196) radius 1.6 projected
  circle A36 centre (-39.9568, -59.168) radius 2.5 projected
  circle A37 centre (-42.8052, -51.6922) radius 1.6 projected
  circle A38 centre (-39.9568, -59.168) radius 2
  point P0 (0, 0)
  dimension "d48" = 4
  constraints: 1 centre point, 1 coincident
  measures "d48" diameter of A38
extrude "Выдавливание17" add sketch "Эскиз20" against normal up to surface (5 mm away) contours A36
sketch "Эскиз21" plane through (0, 0, 0) normal (0, 0, -1) x (-1, 0, 0)
  circle A0 centre (39.9568, -59.168) radius 2 projected
  arc A1 (40.5666, -46.8005) -> (39.6828, -46.7885) centre (39.9568, -59.168) ccw projected
  arc A2 (39.6828, -46.7885) -> (38.5334, -43.9946) centre (28.9908, -49.5535) ccw projected
  arc A3 (38.5334, -43.9946) -> (37.4546, -44.1348) centre (39.9568, -59.168) ccw projected
  arc A4 (37.4546, -44.1348) -> (37.0576, -47.1297) centre (48.1012, -47.07) ccw projected
  arc A5 (37.0576, -47.1297) -> (36.2062, -47.3672) centre (39.9568, -59.168) ccw projected
  arc A6 (36.2062, -47.3672) -> (34.3163, -45.0102) centre (26.7263, -53.0325) ccw projected
  arc A7 (34.3163, -45.0102) -> (33.3206, -45.4487) centre (39.9568, -59.168) ccw projected
  arc A8 (33.3206, -45.4487) -> (33.7834, -48.4341) centre (44.3629, -45.2655) ccw projected
  arc A9 (33.7834, -48.4341) -> (33.0334, -48.9019) centre (39.9568, -59.168) ccw projected
  arc A10 (33.0334, -48.9019) -> (30.556, -47.1729) centre (25.5336, -57.0085) ccw projected
  arc A11 (30.556, -47.1729) -> (29.7243, -47.8741) centre (39.9568, -59.168) ccw projected
  arc A12 (29.7243, -47.8741) -> (31.0094, -50.6082) centre (40.2676, -44.5873) ccw projected
  arc A13 (31.0094, -50.6082) -> (30.4216, -51.2683) centre (39.9568, -59.168) ccw projected
  arc A14 (30.4216, -51.2683) -> (27.5574, -50.3073) centre (25.5094, -61.1594) ccw projected
  arc A15 (27.5574, -50.3073) -> (26.9569, -51.2144) centre (39.9568, -59.168) ccw projected
  arc A16 (26.9569, -51.2144) -> (28.9603, -53.4757) centre (36.1472, -45.0904) ccw projected
  arc A17 (28.9603, -53.4757) -> (28.5822, -54.2747) centre (39.9568, -59.168) ccw projected
  arc A18 (28.5822, -54.2747) -> (25.5633, -54.1595) centre (26.6557, -65.1491) ccw projected
  arc A19 (25.5633, -54.1595) -> (25.2427, -55.1991) centre (39.9568, -59.168) ccw projected
  arc A20 (25.2427, -55.1991) -> (27.802, -56.8043) centre (32.3353, -46.7339) ccw projected
  arc A21 (27.802, -56.8043) -> (27.6644, -57.6775) centre (39.9568, -59.168) ccw projected
  arc A22 (27.6644, -57.6775) -> (24.7353, -58.4175) centre (28.8796, -68.6541) ccw projected
  arc A23 (24.7353, -58.4175) -> (24.7206, -59.5053) centre (39.9568, -59.168) ccw projected
  arc A24 (24.7206, -59.5053) -> (27.6284, -60.3245) centre (29.141, -49.3848) ccw projected
  arc A25 (27.6284, -60.3245) -> (27.7424, -61.201) centre (39.9568, -59.168) ccw projected
  arc A26 (27.7424, -61.201) -> (25.1404, -62.7363) centre (32.0008, -71.3907) ccw projected
  arc A27 (25.1404, -62.7363) -> (25.4328, -63.7842) centre (39.9568, -59.168) ccw projected
  arc A28 (25.4328, -63.7842) -> (28.4537, -63.7509) centre (26.8229, -52.8283) ccw projected
  arc A29 (28.4537, -63.7509) -> (48.6356, -68) centre (39.9568, -59.168) ccw projected
  line L0 (48.6356, -68) -> (71.6748, -50.2404) projected
  line L1 (71.6748, -50.2404) -> (73.2914, -45.6377) projected
  line L2 (73.2914, -45.6377) -> (74.8978, -22.7778) projected
  line L3 (74.8978, -22.7778) -> (67.7849, -22.278) projected
  line L4 (67.7849, -22.278) -> (66.4131, -41.803) projected
  line L5 (66.4131, -41.803) -> (65.4189, -44.6336) projected
  line L6 (65.4189, -44.6336) -> (48.2799, -50) projected
  arc A30 (48.2799, -50) -> (43.1816, -47.2128) centre (39.9568, -59.168) ccw projected
  arc A31 (43.1816, -47.2128) -> (42.8659, -44.2082) centre (32.1437, -46.8535) ccw projected
  arc A32 (42.8659, -44.2082) -> (41.7913, -44.0388) centre (39.9568, -59.168) ccw projected
  arc A33 (41.7913, -44.0388) -> (40.5666, -46.8005) centre (51.1797, -49.8545) ccw projected
  circle A34 centre (42.8052, -51.6922) radius 1.6 projected
  circle A35 centre (32.4811, -56.3196) radius 1.6 projected
  circle A36 centre (37.1084, -66.6437) radius 1.6 projected
  circle A37 centre (47.4326, -62.0164) radius 1.6 projected
  arc A38 (28.4373, -63.7097) -> (28.7906, -64.5199) centre (39.9568, -59.168) ccw
  arc A39 (28.7906, -64.5199) -> (26.7188, -66.7186) centre (35.7166, -73.122) ccw
  arc A40 (26.7188, -66.7186) -> (27.2911, -67.6437) centre (39.9568, -59.168) ccw
  arc A41 (27.2911, -67.6437) -> (30.1835, -66.7711) centre (25.5774, -56.7338) ccw
  arc A42 (30.1835, -66.7711) -> (30.7508, -67.449) centre (39.9568, -59.168) ccw
  arc A43 (30.7508, -67.449) -> (29.3822, -70.1423) centre (39.8196, -73.7513) ccw
  arc A44 (29.3822, -70.1423) -> (30.1921, -70.8687) centre (39.9568, -59.168) ccw
  arc A45 (30.1921, -70.8687) -> (32.7214, -69.2166) centre (25.4741, -60.8835) ccw
  arc A46 (32.7214, -69.2166) -> (33.4567, -69.7072) centre (39.9568, -59.168) ccw
  arc A47 (33.4567, -69.7072) -> (32.9024, -72.677) centre (43.9338, -73.1993) ccw
  arc A48 (32.9024, -72.677) -> (33.8841, -73.1458) centre (39.9568, -59.168) ccw
  arc A49 (33.8841, -73.1458) -> (35.8455, -70.848) centre (26.5441, -64.8943) ccw
  arc A50 (35.8455, -70.848) -> (36.6892, -71.1116) centre (39.9568, -59.168) ccw
  arc A51 (36.6892, -71.1116) -> (36.9941, -74.1172) centre (47.7258, -71.5105) ccw
  arc A52 (36.9941, -74.1172) -> (38.0681, -74.2905) centre (39.9568, -59.168) ccw
  arc A53 (38.0681, -74.2905) -> (39.3027, -71.5332) centre (28.7006, -68.4411) ccw
  arc A54 (39.3027, -71.5332) -> (40.1865, -71.5484) centre (39.9568, -59.168) ccw
  arc A55 (40.1865, -71.5484) -> (41.3258, -74.3464) centre (50.8883, -68.8217) ccw
  arc A56 (41.3258, -74.3464) -> (42.4051, -74.21) centre (39.9568, -59.168) ccw
  arc A57 (42.4051, -74.21) -> (42.8129, -71.2166) centre (31.7691, -71.2367) ccw
  arc A58 (42.8129, -71.2166) -> (43.6651, -70.9822) centre (39.9568, -59.168) ccw
  arc A59 (43.6651, -70.9822) -> (45.5466, -73.3459) centre (53.1653, -65.3509) ccw
  arc A60 (45.5466, -73.3459) -> (46.5438, -72.911) centre (39.9568, -59.168) ccw
  arc A61 (46.5438, -72.911) -> (46.0917, -69.9239) centre (35.501, -73.0546) ccw
  arc A62 (46.0917, -69.9239) -> (46.8434, -69.4589) centre (39.9568, -59.168) ccw
  point P0 (0, 0)
  point P1 (39.5938, -73.7475)
  point P2 (46.0917, -69.9239)
  point P3 (43.6651, -70.9822)
  point P4 (42.8129, -71.2166)
  point P5 (40.1865, -71.5484)
  point P6 (39.3027, -71.5332)
  point P7 (36.6892, -71.1116)
  point P8 (33.4567, -69.7072)
  point P9 (32.7214, -69.2166)
  point P10 (30.7508, -67.449)
  point P11 (30.1835, -66.7711)
  point P12 (28.7906, -64.5199)
  constraints: 50 point on circle, 25 centre point
extrude "Выдавливание18" add sketch "Эскиз21" against normal up to surface (5 mm away) contours A49 A48 A47 A29 | A45 A44 A43 A29 | A41 A40 A39 A29
sketch "Эскиз22" plane through (0, 0, 5) normal (0, 0, 1) x (1, 0, 0)
  circle A0 centre (-39.9568, -59.168) radius 2 projected
  arc A1 (-38.5334, -43.9946) -> (-39.6828, -46.7885) centre (-28.9908, -49.5535) ccw projected
  arc A2 (-39.6828, -46.7885) -> (-40.5666, -46.8005) centre (-39.9568, -59.168) ccw projected
  arc A3 (-40.5666, -46.8005) -> (-41.7913, -44.0388) centre (-51.1797, -49.8545) ccw projected
  arc A4 (-41.7913, -44.0388) -> (-42.8659, -44.2082) centre (-39.9568, -59.168) ccw projected
  arc A5 (-42.8659, -44.2082) -> (-43.1816, -47.2128) centre (-32.1437, -46.8535) ccw projected
  arc A6 (-43.1816, -47.2128) -> (-48.2799, -50) centre (-39.9568, -59.168) ccw projected
  line L0 (-48.2799, -50) -> (-65.4189, -44.6336) projected
  line L1 (-65.4189, -44.6336) -> (-66.4131, -41.803) projected
  line L2 (-66.4131, -41.803) -> (-67.7849, -22.278) projected
  line L3 (-67.7849, -22.278) -> (-74.8978, -22.7778) projected
  line L4 (-74.8978, -22.7778) -> (-73.2914, -45.6377) projected
  line L5 (-73.2914, -45.6377) -> (-71.6748, -50.2404) projected
  line L6 (-71.6748, -50.2404) -> (-48.6356, -68) projected
  arc A7 (-48.6356, -68) -> (-35.8455, -70.848) centre (-39.9568, -59.168) ccw projected
  arc A8 (-35.8455, -70.848) -> (-33.8841, -73.1458) centre (-26.5441, -64.8943) ccw projected
  arc A9 (-33.8841, -73.1458) -> (-32.9024, -72.677) centre (-39.9568, -59.168) ccw projected
  arc A10 (-32.9024, -72.677) -> (-33.4567, -69.7072) centre (-43.9338, -73.1993) ccw projected
  arc A11 (-33.4567, -69.7072) -> (-32.7214, -69.2166) centre (-39.9568, -59.168) ccw projected
  arc A12 (-32.7214, -69.2166) -> (-30.1921, -70.8687) centre (-25.4741, -60.8835) ccw projected
  arc A13 (-30.1921, -70.8687) -> (-29.3822, -70.1423) centre (-39.9568, -59.168) ccw projected
  arc A14 (-29.3822, -70.1423) -> (-30.7508, -67.449) centre (-39.8196, -73.7513) ccw projected
  arc A15 (-30.7508, -67.449) -> (-30.1835, -66.7711) centre (-39.9568, -59.168) ccw projected
  arc A16 (-30.1835, -66.7711) -> (-27.2911, -67.6437) centre (-25.5774, -56.7338) ccw projected
  arc A17 (-27.2911, -67.6437) -> (-26.7188, -66.7186) centre (-39.9568, -59.168) ccw projected
  arc A18 (-26.7188, -66.7186) -> (-28.7906, -64.5199) centre (-35.7166, -73.122) ccw projected
  arc A19 (-28.7906, -64.5199) -> (-28.4537, -63.7509) centre (-39.9568, -59.168) ccw projected
  arc A20 (-28.4537, -63.7509) -> (-25.4328, -63.7842) centre (-26.8229, -52.8283) ccw projected
  arc A21 (-25.4328, -63.7842) -> (-25.1404, -62.7363) centre (-39.9568, -59.168) ccw projected
  arc A22 (-25.1404, -62.7363) -> (-27.7424, -61.201) centre (-32.0008, -71.3907) ccw projected
  arc A23 (-27.7424, -61.201) -> (-27.6284, -60.3245) centre (-39.9568, -59.168) ccw projected
  arc A24 (-27.6284, -60.3245) -> (-24.7206, -59.5053) centre (-29.141, -49.3848) ccw projected
  arc A25 (-24.7206, -59.5053) -> (-24.7353, -58.4175) centre (-39.9568, -59.168) ccw projected
  arc A26 (-24.7353, -58.4175) -> (-27.6644, -57.6775) centre (-28.8796, -68.6541) ccw projected
  arc A27 (-27.6644, -57.6775) -> (-27.802, -56.8043) centre (-39.9568, -59.168) ccw projected
  arc A28 (-27.802, -56.8043) -> (-25.2427, -55.1991) centre (-32.3353, -46.7339) ccw projected
  arc A29 (-25.2427, -55.1991) -> (-25.5633, -54.1595) centre (-39.9568, -59.168) ccw projected
  arc A30 (-25.5633, -54.1595) -> (-28.5822, -54.2747) centre (-26.6557, -65.1491) ccw projected
  arc A31 (-28.5822, -54.2747) -> (-28.9603, -53.4757) centre (-39.9568, -59.168) ccw projected
  arc A32 (-28.9603, -53.4757) -> (-26.9569, -51.2144) centre (-36.1472, -45.0904) ccw projected
  arc A33 (-26.9569, -51.2144) -> (-27.5574, -50.3073) centre (-39.9568, -59.168) ccw projected
  arc A34 (-27.5574, -50.3073) -> (-30.4216, -51.2683) centre (-25.5094, -61.1594) ccw projected
  arc A35 (-30.4216, -51.2683) -> (-31.0094, -50.6082) centre (-39.9568, -59.168) ccw projected
  arc A36 (-31.0094, -50.6082) -> (-29.7243, -47.8741) centre (-40.2676, -44.5873) ccw projected
  arc A37 (-29.7243, -47.8741) -> (-30.556, -47.1729) centre (-39.9568, -59.168) ccw projected
  arc A38 (-30.556, -47.1729) -> (-33.0334, -48.9019) centre (-25.5336, -57.0085) ccw projected
  arc A39 (-33.0334, -48.9019) -> (-33.7834, -48.4341) centre (-39.9568, -59.168) ccw projected
  arc A40 (-33.7834, -48.4341) -> (-33.3206, -45.4487) centre (-44.3629, -45.2655) ccw projected
  arc A41 (-33.3206, -45.4487) -> (-34.3163, -45.0102) centre (-39.9568, -59.168) ccw projected
  arc A42 (-34.3163, -45.0102) -> (-36.2062, -47.3672) centre (-26.7263, -53.0325) ccw projected
  arc A43 (-36.2062, -47.3672) -> (-37.0576, -47.1297) centre (-39.9568, -59.168) ccw projected
  arc A44 (-37.0576, -47.1297) -> (-37.4546, -44.1348) centre (-48.1012, -47.07) ccw projected
  arc A45 (-37.4546, -44.1348) -> (-38.5334, -43.9946) centre (-39.9568, -59.168) ccw projected
  circle A46 centre (-47.4326, -62.0164) radius 1.6 projected
  circle A47 centre (-37.1084, -66.6437) radius 1.6 projected
  circle A48 centre (-32.4811, -56.3196) radius 1.6 projected
  circle A49 centre (-42.8052, -51.6922) radius 1.6 projected
  line L7 (-33.4567, -69.7072) -> (-32.0008, -74.4957)
  line L8 (-32.0008, -74.4957) -> (-33, -75)
  line L9 (-33, -75) -> (-35.8455, -70.848)
  point P0 (0, 0)
  point P1 (-35.453, -71.4208)
  point P2 (-33.286, -70.2687)
  constraints: 6 end point
extrude "Выдавливание19" add sketch "Эскиз22" against normal up to surface (5 mm away)
sketch "Эскиз23" plane through (0, 0, 5) normal (0, 0, 1) x (1, 0, 0)
  circle A0 centre (-39.9568, -59.168) radius 2 projected
  arc A1 (-38.5334, -43.9946) -> (-39.6828, -46.7885) centre (-28.9908, -49.5535) ccw projected
  arc A2 (-39.6828, -46.7885) -> (-40.5666, -46.8005) centre (-39.9568, -59.168) ccw projected
  arc A3 (-40.5666, -46.8005) -> (-41.7913, -44.0388) centre (-51.1797, -49.8545) ccw projected
  arc A4 (-41.7913, -44.0388) -> (-42.8659, -44.2082) centre (-39.9568, -59.168) ccw projected
  arc A5 (-42.8659, -44.2082) -> (-43.1816, -47.2128) centre (-32.1437, -46.8535) ccw projected
  arc A6 (-43.1816, -47.2128) -> (-48.2799, -50) centre (-39.9568, -59.168) ccw projected
  line L0 (-48.2799, -50) -> (-65.4189, -44.6336) projected
  line L1 (-65.4189, -44.6336) -> (-66.4131, -41.803) projected
  line L2 (-66.4131, -41.803) -> (-67.7849, -22.278) projected
  line L3 (-67.7849, -22.278) -> (-74.8978, -22.7778) projected
  line L4 (-74.8978, -22.7778) -> (-73.2914, -45.6377) projected
  line L5 (-73.2914, -45.6377) -> (-71.6748, -50.2404) projected
  line L6 (-71.6748, -50.2404) -> (-48.6356, -68) projected
  arc A7 (-48.6356, -68) -> (-35.8455, -70.848) centre (-39.9568, -59.168) ccw projected
  arc A8 (-35.8455, -70.848) -> (-35.453, -71.4208) centre (-26.5441, -64.8943) ccw projected
  line L7 (-35.453, -71.4208) -> (-33, -75) projected
  line L8 (-33, -75) -> (-32.0008, -74.4957) projected
  line L9 (-32.0008, -74.4957) -> (-33.286, -70.2687) projected
  arc A9 (-33.286, -70.2687) -> (-33.4567, -69.7072) centre (-43.9338, -73.1993) ccw projected
  arc A10 (-33.4567, -69.7072) -> (-32.7214, -69.2166) centre (-39.9568, -59.168) ccw projected
  arc A11 (-32.7214, -69.2166) -> (-30.1921, -70.8687) centre (-25.4741, -60.8835) ccw projected
  arc A12 (-30.1921, -70.8687) -> (-29.3822, -70.1423) centre (-39.9568, -59.168) ccw projected
  arc A13 (-29.3822, -70.1423) -> (-30.7508, -67.449) centre (-39.8196, -73.7513) ccw projected
  arc A14 (-30.7508, -67.449) -> (-30.1835, -66.7711) centre (-39.9568, -59.168) ccw projected
  arc A15 (-30.1835, -66.7711) -> (-27.2911, -67.6437) centre (-25.5774, -56.7338) ccw projected
  arc A16 (-27.2911, -67.6437) -> (-26.7188, -66.7186) centre (-39.9568, -59.168) ccw projected
  arc A17 (-26.7188, -66.7186) -> (-28.7906, -64.5199) centre (-35.7166, -73.122) ccw projected
  arc A18 (-28.7906, -64.5199) -> (-28.4537, -63.7509) centre (-39.9568, -59.168) ccw projected
  arc A19 (-28.4537, -63.7509) -> (-25.4328, -63.7842) centre (-26.8229, -52.8283) ccw projected
  arc A20 (-25.4328, -63.7842) -> (-25.1404, -62.7363) centre (-39.9568, -59.168) ccw projected
  arc A21 (-25.1404, -62.7363) -> (-27.7424, -61.201) centre (-32.0008, -71.3907) ccw projected
  arc A22 (-27.7424, -61.201) -> (-27.6284, -60.3245) centre (-39.9568, -59.168) ccw projected
  arc A23 (-27.6284, -60.3245) -> (-24.7206, -59.5053) centre (-29.141, -49.3848) ccw projected
  arc A24 (-24.7206, -59.5053) -> (-24.7353, -58.4175) centre (-39.9568, -59.168) ccw projected
  arc A25 (-24.7353, -58.4175) -> (-27.6644, -57.6775) centre (-28.8796, -68.6541) ccw projected
  arc A26 (-27.6644, -57.6775) -> (-27.802, -56.8043) centre (-39.9568, -59.168) ccw projected
  arc A27 (-27.802, -56.8043) -> (-25.2427, -55.1991) centre (-32.3353, -46.7339) ccw projected
  arc A28 (-25.2427, -55.1991) -> (-25.5633, -54.1595) centre (-39.9568, -59.168) ccw projected
  arc A29 (-25.5633, -54.1595) -> (-28.5822, -54.2747) centre (-26.6557, -65.1491) ccw projected
  arc A30 (-28.5822, -54.2747) -> (-28.9603, -53.4757) centre (-39.9568, -59.168) ccw projected
  arc A31 (-28.9603, -53.4757) -> (-26.9569, -51.2144) centre (-36.1472, -45.0904) ccw projected
  arc A32 (-26.9569, -51.2144) -> (-27.5574, -50.3073) centre (-39.9568, -59.168) ccw projected
  arc A33 (-27.5574, -50.3073) -> (-30.4216, -51.2683) centre (-25.5094, -61.1594) ccw projected
  arc A34 (-30.4216, -51.2683) -> (-31.0094, -50.6082) centre (-39.9568, -59.168) ccw projected
  arc A35 (-31.0094, -50.6082) -> (-29.7243, -47.8741) centre (-40.2676, -44.5873) ccw projected
  arc A36 (-29.7243, -47.8741) -> (-30.556, -47.1729) centre (-39.9568, -59.168) ccw projected
  arc A37 (-30.556, -47.1729) -> (-33.0334, -48.9019) centre (-25.5336, -57.0085) ccw projected
  arc A38 (-33.0334, -48.9019) -> (-33.7834, -48.4341) centre (-39.9568, -59.168) ccw projected
  arc A39 (-33.7834, -48.4341) -> (-33.3206, -45.4487) centre (-44.3629, -45.2655) ccw projected
  arc A40 (-33.3206, -45.4487) -> (-34.3163, -45.0102) centre (-39.9568, -59.168) ccw projected
  arc A41 (-34.3163, -45.0102) -> (-36.2062, -47.3672) centre (-26.7263, -53.0325) ccw projected
  arc A42 (-36.2062, -47.3672) -> (-37.0576, -47.1297) centre (-39.9568, -59.168) ccw projected
  arc A43 (-37.0576, -47.1297) -> (-37.4546, -44.1348) centre (-48.1012, -47.07) ccw projected
  arc A44 (-37.4546, -44.1348) -> (-38.5334, -43.9946) centre (-39.9568, -59.168) ccw projected
  circle A45 centre (-47.4326, -62.0164) radius 1.6 projected
  circle A46 centre (-37.1084, -66.6437) radius 1.6 projected
  circle A47 centre (-32.4811, -56.3196) radius 1.6 projected
  circle A48 centre (-42.8052, -51.6922) radius 1.6 projected
  line L10 (-74.962, -41.6455) -> (-75.9562, -38.8149)
  line L11 (-75.9562, -38.8149) -> (-77.328, -19.2899)
  line L12 (-77.328, -19.2899) -> (-84.4409, -19.7898)
  line L13 (-84.4409, -19.7898) -> (-82.8346, -42.6496)
  line L14 (-82.8346, -42.6496) -> (-81.2179, -47.2523)
  line L15 (-65.4189, -44.6336) -> (-74.962, -41.6455)
  line L16 (-81.2179, -47.2523) -> (-48.6356, -68)
  point P0 (0, 0)
  point P1 (-73.5407, -42.0905)
  dimension "d55" = 10
  constraints: 14 end point, 1 collinear
  measures "d55" distance of L0.end L15.end
extrude "Выдавливание20" add sketch "Эскиз23" against normal up to surface (5 mm away) contours L4 L5 L6 L16 L14 L13 L12 L11 L10 L15
sketch "Эскиз24" plane through (0, 0, 5) normal (0, 0, 1) x (1, 0, 0)
  circle A0 centre (-39.9568, -59.168) radius 2 projected
  arc A1 (-38.5334, -43.9946) -> (-39.6828, -46.7885) centre (-28.9908, -49.5535) ccw projected
  arc A2 (-39.6828, -46.7885) -> (-40.5666, -46.8005) centre (-39.9568, -59.168) ccw projected
  arc A3 (-40.5666, -46.8005) -> (-41.7913, -44.0388) centre (-51.1797, -49.8545) ccw projected
  arc A4 (-41.7913, -44.0388) -> (-42.8659, -44.2082) centre (-39.9568, -59.168) ccw projected
  arc A5 (-42.8659, -44.2082) -> (-43.1816, -47.2128) centre (-32.1437, -46.8535) ccw projected
  arc A6 (-43.1816, -47.2128) -> (-48.2799, -50) centre (-39.9568, -59.168) ccw projected
  line L0 (-48.2799, -50) -> (-65.4189, -44.6336) projected
  line L1 (-65.4189, -44.6336) -> (-66.4131, -41.803) projected
  line L2 (-66.4131, -41.803) -> (-67.7849, -22.278) projected
  line L3 (-67.7849, -22.278) -> (-74.8978, -22.7778) projected
  line L4 (-74.8978, -22.7778) -> (-73.5407, -42.0905) projected
  line L5 (-73.5407, -42.0905) -> (-74.962, -41.6455) projected
  line L6 (-74.962, -41.6455) -> (-75.9562, -38.8149) projected
  line L7 (-75.9562, -38.8149) -> (-77.328, -19.2899) projected
  line L8 (-77.328, -19.2899) -> (-84.4409, -19.7898) projected
  line L9 (-84.4409, -19.7898) -> (-82.8346, -42.6496) projected
  line L10 (-82.8346, -42.6496) -> (-81.2179, -47.2523) projected
  line L11 (-81.2179, -47.2523) -> (-48.6356, -68) projected
  arc A7 (-48.6356, -68) -> (-35.8455, -70.848) centre (-39.9568, -59.168) ccw projected
  arc A8 (-35.8455, -70.848) -> (-35.453, -71.4208) centre (-26.5441, -64.8943) ccw projected
  line L12 (-35.453, -71.4208) -> (-33, -75) projected
  line L13 (-33, -75) -> (-32.0008, -74.4957) projected
  line L14 (-32.0008, -74.4957) -> (-33.286, -70.2687) projected
  arc A9 (-33.286, -70.2687) -> (-33.4567, -69.7072) centre (-43.9338, -73.1993) ccw projected
  arc A10 (-33.4567, -69.7072) -> (-32.7214, -69.2166) centre (-39.9568, -59.168) ccw projected
  arc A11 (-32.7214, -69.2166) -> (-30.1921, -70.8687) centre (-25.4741, -60.8835) ccw projected
  arc A12 (-30.1921, -70.8687) -> (-29.3822, -70.1423) centre (-39.9568, -59.168) ccw projected
  arc A13 (-29.3822, -70.1423) -> (-30.7508, -67.449) centre (-39.8196, -73.7513) ccw projected
  arc A14 (-30.7508, -67.449) -> (-30.1835, -66.7711) centre (-39.9568, -59.168) ccw projected
  arc A15 (-30.1835, -66.7711) -> (-27.2911, -67.6437) centre (-25.5774, -56.7338) ccw projected
  arc A16 (-27.2911, -67.6437) -> (-26.7188, -66.7186) centre (-39.9568, -59.168) ccw projected
  arc A17 (-26.7188, -66.7186) -> (-28.7906, -64.5199) centre (-35.7166, -73.122) ccw projected
  arc A18 (-28.7906, -64.5199) -> (-28.4537, -63.7509) centre (-39.9568, -59.168) ccw projected
  arc A19 (-28.4537, -63.7509) -> (-25.4328, -63.7842) centre (-26.8229, -52.8283) ccw projected
  arc A20 (-25.4328, -63.7842) -> (-25.1404, -62.7363) centre (-39.9568, -59.168) ccw projected
  arc A21 (-25.1404, -62.7363) -> (-27.7424, -61.201) centre (-32.0008, -71.3907) ccw projected
  arc A22 (-27.7424, -61.201) -> (-27.6284, -60.3245) centre (-39.9568, -59.168) ccw projected
  arc A23 (-27.6284, -60.3245) -> (-24.7206, -59.5053) centre (-29.141, -49.3848) ccw projected
  arc A24 (-24.7206, -59.5053) -> (-24.7353, -58.4175) centre (-39.9568, -59.168) ccw projected
  arc A25 (-24.7353, -58.4175) -> (-27.6644, -57.6775) centre (-28.8796, -68.6541) ccw projected
  arc A26 (-27.6644, -57.6775) -> (-27.802, -56.8043) centre (-39.9568, -59.168) ccw projected
  arc A27 (-27.802, -56.8043) -> (-25.2427, -55.1991) centre (-32.3353, -46.7339) ccw projected
  arc A28 (-25.2427, -55.1991) -> (-25.5633, -54.1595) centre (-39.9568, -59.168) ccw projected
  arc A29 (-25.5633, -54.1595) -> (-28.5822, -54.2747) centre (-26.6557, -65.1491) ccw projected
  arc A30 (-28.5822, -54.2747) -> (-28.9603, -53.4757) centre (-39.9568, -59.168) ccw projected
  arc A31 (-28.9603, -53.4757) -> (-26.9569, -51.2144) centre (-36.1472, -45.0904) ccw projected
  arc A32 (-26.9569, -51.2144) -> (-27.5574, -50.3073) centre (-39.9568, -59.168) ccw projected
  arc A33 (-27.5574, -50.3073) -> (-30.4216, -51.2683) centre (-25.5094, -61.1594) ccw projected
  arc A34 (-30.4216, -51.2683) -> (-31.0094, -50.6082) centre (-39.9568, -59.168) ccw projected
  arc A35 (-31.0094, -50.6082) -> (-29.7243, -47.8741) centre (-40.2676, -44.5873) ccw projected
  arc A36 (-29.7243, -47.8741) -> (-30.556, -47.1729) centre (-39.9568, -59.168) ccw projected
  arc A37 (-30.556, -47.1729) -> (-33.0334, -48.9019) centre (-25.5336, -57.0085) ccw projected
  arc A38 (-33.0334, -48.9019) -> (-33.7834, -48.4341) centre (-39.9568, -59.168) ccw projected
  arc A39 (-33.7834, -48.4341) -> (-33.3206, -45.4487) centre (-44.3629, -45.2655) ccw projected
  arc A40 (-33.3206, -45.4487) -> (-34.3163, -45.0102) centre (-39.9568, -59.168) ccw projected
  arc A41 (-34.3163, -45.0102) -> (-36.2062, -47.3672) centre (-26.7263, -53.0325) ccw projected
  arc A42 (-36.2062, -47.3672) -> (-37.0576, -47.1297) centre (-39.9568, -59.168) ccw projected
  arc A43 (-37.0576, -47.1297) -> (-37.4546, -44.1348) centre (-48.1012, -47.07) ccw projected
  arc A44 (-37.4546, -44.1348) -> (-38.5334, -43.9946) centre (-39.9568, -59.168) ccw projected
  circle A45 centre (-47.4326, -62.0164) radius 1.6 projected
  circle A46 centre (-37.1084, -66.6437) radius 1.6 projected
  circle A47 centre (-32.4811, -56.3196) radius 1.6 projected
  circle A48 centre (-42.8052, -51.6922) radius 1.6 projected
  line L15 (-73.5407, -42.0905) -> (-65.4189, -44.6336)
  point P0 (0, 0)
  constraints: 2 end point, 1 collinear
extrude "Выдавливание21" cut sketch "Эскиз24" against normal blind 10 contours L15 L4 L3 L2 L1
